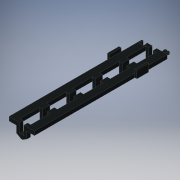
# Autodesk Inventor part: PRO10315 Rolle fuer Rollenleiste 178
Saved by Autodesk Inventor 2019 (Build 230136000, 136)
## iProperties
Created: 2023-08-22
Part Number: PRO10315 Rolle fuer Rollenleiste 178
Material: Generic
Catalog Web Link: www.cadenas.de
Description: PRO10315-Rolle fuer Rollenleiste
Vendor: ROBOTUNITS
Document SubType Name: Modeling
Designer: psAdmin
Manufacturer: ROBOTUNITS
Mass: 26.2793 g
Surface Area: 164.045 cm^2
Volume: 26.2793 cm^3
Density: 1 g/cm^3
Appearance: PSOLRGB-127-135-137
Category: PARTsolutions
Company: ROBOTUNITS
Title: PRO10315 Rolle fuer Rollenleiste 178
Author: Cadenas PARTsolutions
Comments: Rolle fuer Rollenleiste
PSOL_IDENT_0: {$CADENAS_DATA/23d-libs/robotunits/mbs_pickstar/parts_materialbereitstellungssystem/pro_10315.prj},2
PSOL_IDENT_1: 16 {VTYP=3D},{NB=PRO10315 Rolle fuer Rollenleiste 178},{LINA=PRO10315 Rolle fuer Rollenleiste 178},{
PSOL_IDENT_2: NN=PRO10315},{DATE=25.04.2023 06:51:54},{GEOMDATE=14.02.2017 14:53:00},{VERSION=},{LINEID=10},{WBVAR=
PSOL_IDENT_3: L},{WBNUMERIC=L}  {NB=PRO10315 Rolle fuer Rollenleiste 178},{LINA=PRO10315 Rolle fuer Rollenleiste 1
PSOL_IDENT_4: 78},{KT=DUMMY},{L=178},{LX=0178},{LXX=250,[45:250]},{B=39.500},{L2=0}
NB: PRO10315 Rolle fuer Rollenleiste 178
NN: PRO10315
NT: Rolle fuer Rollenleiste
NBSYN: PRO10315 Rolle fuer Rollenleiste $L.
LINA: PRO10315 Rolle fuer Rollenleiste 178
CATALOG: Robotunits
L: 178
B: 39.5
SUPPLIER: ROBOTUNITS
ARTICLENO: PRO10315 Rolle fuer Rollenleiste 178
BOMINFO: PRO10315 Rolle fuer Rollenleiste 178
CREATOR: CADENAS GmbH
Autodesk Inventor part; units mm, degrees
ref_plane "YZ Plane" through (0, 0, 0) normal (1, 0, 0) x (0, 1, 0)
ref_plane "XZ Plane" through (0, 0, 0) normal (0, 1, 0) x (-1, 0, 0)
ref_plane "XY Plane" through (0, 0, 0) normal (0, 0, 1) x (1, 0, 0)
sketch "Sketch_1" plane through (0, 0, 0) normal (0, 0, 1) x (1, 0, 0)
  line L0 (-17, 17.82) -> (-17, 12.62)
  line L1 (-17, 12.62) -> (-6.9, 12.62)
  line L2 (-6.9, 12.62) -> (-6.9, 3.4641)
  line L3 (-6.9, 3.4641) -> (-0.9, 0)
  line L4 (-0.9, 0) -> (0.9, 0)
  line L5 (0.9, 0) -> (6.9, 3.4641)
  line L6 (6.9, 3.4641) -> (6.9, 12.62)
  line L7 (6.9, 12.62) -> (17, 12.62)
  line L8 (17, 12.62) -> (17, 17.82)
  line L9 (17, 17.82) -> (3, 17.82)
  line L10 (3, 17.82) -> (3, 5.67)
  line L11 (3, 5.67) -> (-3, 5.67)
  line L12 (-3, 5.67) -> (-3, 17.82)
  line L13 (-3, 17.82) -> (-17, 17.82)
  constraints: 28 end point
extrude "Extrusion1" add sketch "Sketch_1" along normal blind 178
sketch "Sketch_9" plane through (0, 0, 0) normal (0, 1, 0) x (-1, 0, 0)
  line L0 (7.12, 4.62) -> (7.12, 30.82)
  line L1 (7.12, 30.82) -> (-7.12, 30.82)
  line L2 (-7.12, 30.82) -> (-7.12, 4.62)
  line L3 (-7.12, 4.62) -> (7.12, 4.62)
  constraints: 8 end point
extrude "Extrusion2" cut sketch "Sketch_9" along normal blind 25
sketch "Sketch_2" plane through (0, 0, 0) normal (0, 1, 0) x (-1, 0, 0)
  line L0 (7.12, 40.33) -> (7.12, 66.53)
  line L1 (7.12, 66.53) -> (-7.12, 66.53)
  line L2 (-7.12, 66.53) -> (-7.12, 40.33)
  line L3 (-7.12, 40.33) -> (7.12, 40.33)
  constraints: 8 end point
extrude "Extrusion3" cut sketch "Sketch_2" along normal blind 25
sketch "Sketch_3" plane through (0, 0, 0) normal (0, 1, 0) x (-1, 0, 0)
  line L0 (7.12, 76.04) -> (7.12, 102.24)
  line L1 (7.12, 102.24) -> (-7.12, 102.24)
  line L2 (-7.12, 102.24) -> (-7.12, 76.04)
  line L3 (-7.12, 76.04) -> (7.12, 76.04)
  constraints: 8 end point
extrude "Extrusion4" cut sketch "Sketch_3" along normal blind 25
sketch "Sketch_4" plane through (0, 0, 0) normal (0, 1, 0) x (-1, 0, 0)
  line L0 (7.12, 111.21) -> (7.12, 137.41)
  line L1 (7.12, 137.41) -> (-7.12, 137.41)
  line L2 (-7.12, 137.41) -> (-7.12, 111.21)
  line L3 (-7.12, 111.21) -> (7.12, 111.21)
  constraints: 8 end point
extrude "Extrusion5" cut sketch "Sketch_4" along normal blind 25
sketch "Sketch_5" plane through (0, 0, 0) normal (0, 1, 0) x (-1, 0, 0)
  line L0 (7.12, 146.92) -> (7.12, 173.12)
  line L1 (7.12, 173.12) -> (-7.12, 173.12)
  line L2 (-7.12, 173.12) -> (-7.12, 146.92)
  line L3 (-7.12, 146.92) -> (7.12, 146.92)
  constraints: 8 end point
extrude "Extrusion6" cut sketch "Sketch_5" along normal blind 25
sketch "Sketch_10" plane through (17, 17.82, 0) normal (0, 1, 0) x (-1, 0, 0)
  line L0 (1.15, -3.5) -> (1.95, -5)
  line L1 (1.95, -5) -> (3.75, -5)
  line L2 (3.75, -5) -> (3.75, -0.75)
  arc A0 (4.5, 0) -> (3.75, -0.75) centre (4.5, -0.75) ccw
  arc A1 (5.25, -0.75) -> (4.5, 0) centre (4.5, -0.75) ccw
  line L3 (5.25, -0.75) -> (5.25, -5)
  line L4 (5.25, -5) -> (7.05, -5)
  line L5 (7.05, -5) -> (7.85, -3.5)
  line L6 (7.85, -3.5) -> (7.05, -2)
  line L7 (7.05, -2) -> (7.05, 0.5)
  line L8 (7.05, 0.5) -> (1.95, 0.5)
  line L9 (1.95, 0.5) -> (1.95, -2)
  line L10 (1.95, -2) -> (1.15, -3.5)
  constraints: 22 end point, 4 point on circle, 2 centre point
extrude "Extrusion7" add sketch "Sketch_10" against normal blind 2.7
sketch "Sketch_12" plane through (17, 17.82, 0) normal (0, 1, 0) x (-1, 0, 0)
  line L0 (26.3, 5.6) -> (26.3, 2.5)
  line L1 (26.3, 2.5) -> (26.8, 1.6)
  line L2 (26.8, 1.6) -> (26.8, 0)
  line L3 (26.8, 0) -> (32.2, 0)
  line L4 (32.2, 0) -> (32.2, 1.6)
  line L5 (32.2, 1.6) -> (32.7, 2.5)
  line L6 (32.7, 2.5) -> (32.7, 5.6)
  line L7 (32.7, 5.6) -> (26.3, 5.6)
  constraints: 16 end point
extrude "Extrusion8" cut sketch "Sketch_12" against normal blind 6
sketch "Sketch_16" plane through (-17, 12.62, 0) normal (-1, 0, 0) x (0, 0, 1)
  line L0 (27.9, 10) -> (27.9, 0)
  line L1 (27.9, 0) -> (43.3, 0)
  line L2 (43.3, 0) -> (43.3, 10)
  line L3 (43.3, 10) -> (27.9, 10)
  constraints: 8 end point
extrude "Extrusion9" add sketch "Sketch_16" along normal blind 2.75
sketch "Sketch_14" plane through (17, 17.82, 0) normal (1, 0, 0) x (0, 0, 1)
  line L0 (27.9, -4.8) -> (43.3, -4.8)
  line L1 (43.3, -4.8) -> (43.3, 5.2)
  line L2 (43.3, 5.2) -> (27.9, 5.2)
  line L3 (27.9, 5.2) -> (27.9, -4.8)
  constraints: 8 end point
extrude "Extrusion10" add sketch "Sketch_14" along normal blind 2.75
ref_plane "p1_XY" through (0, 0, 0) normal (0, 1, 0) x (1, 0, 0)
ref_plane "p1_YZ" through (0, 0, 0) normal (1, 0, 0) x (0, 0, -1)
ref_plane "p1_ZX" through (0, 0, 0) normal (0, 0, -1) x (0, 1, 0)
body "Solid1"
